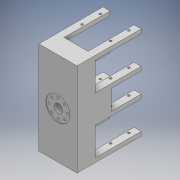
# Autodesk Inventor part: shoulder_5
Saved by Autodesk Inventor 2018 (Build 220112000, 112)
## iProperties
Created: 2020-10-13
Part Number: shoulder_5
Material: 일반
Document SubType Name: Sheet Metal
Designer: j3jjj
Density: 1 g/cm^3
Sheet Metal Rule: 기본값_mm
Appearance: 기본값
Author: j3jjj
Autodesk Inventor part; units mm, degrees
ref_plane "YZ Plane" through (0, 0, 0) normal (1, 0, 0) x (0, 1, 0)
ref_plane "XZ Plane" through (0, 0, 0) normal (0, 1, 0) x (-1, 0, 0)
ref_plane "XY Plane" through (0, 0, 0) normal (0, 0, 1) x (1, 0, 0)
sketch "스케치1" plane through (0, 0, 0) normal (0, 1, 0) x (-1, 0, 0)
  line L0 (23, -56) -> (-23, -56)
  line L1 (-23, -56) -> (-23, 56)
  line L2 (-23, 56) -> (23, 56)
  line L3 (23, 56) -> (23, -56)
  point P0 (0, 0)
  dimension "d0" = 112
  dimension "d1" = 56
  dimension "d2" = 46
  dimension "d3" = 23
  constraints: 8 end point, 2 parallel, 1 horizontal, 1 perpendicular
  measures "d0" distance between parallel lines of L0 L2
  measures "d1" distance from line of point (0, 0) L2
  measures "d2" distance between parallel lines of L1 L3
  measures "d3" distance from line of point (0, 0) L3
extrude "돌출1" add sketch "스케치1" along normal blind 16.1
sketch "스케치2" plane through (0, 0, 0) normal (0, -1, 0) x (1, 0, 0)
  circle A0 centre (0, 0) radius 14.52
  dimension "d6" = 29.04
  constraints: 1 centre point, 1 coincident
  measures "d6" diameter of A0
extrude "돌출2" cut sketch "스케치2" against normal blind 0.5
sketch "스케치3" plane through (0, 0.5, 0) normal (0, -1, 0) x (1, 0, 0)
  circle A0 centre (0, 0) radius 5.075
  circle A1 centre (0, 11) radius 1.25
  circle A2 centre (-7.7782, 7.7782) radius 1.25
  circle A3 centre (-11, 0) radius 1.25
  circle A4 centre (-7.7782, -7.7782) radius 1.25
  circle A5 centre (0, -11) radius 1.25
  circle A6 centre (7.7782, -7.7782) radius 1.25
  circle A7 centre (11, 0) radius 1.25
  circle A8 centre (7.7782, 7.7782) radius 1.25
  dimension "d9" = 10.15
  dimension "d10" = 2.5
  dimension "d11" = 11
  dimension "d14" = 360
  constraints: 9 centre point, 1 coincident, 17 other
  measures "d9" diameter of A0
  measures "d10" diameter of A1
  measures "d11" distance of point (0, 0) A1.centre
extrude "돌출3" cut sketch "스케치3" against normal blind 30
sketch "스케치4" plane through (0, 16.1, 0) normal (0, 1, 0) x (1, 0, 0)
  circle A0 centre (0, -11) radius 1.25 projected
  circle A1 centre (0, -11) radius 3
  circle A2 centre (7.7782, -7.7782) radius 3
  circle A3 centre (11, 0) radius 3
  circle A4 centre (7.7782, 7.7782) radius 3
  circle A5 centre (0, 11) radius 3
  circle A6 centre (-7.7782, 7.7782) radius 3
  circle A7 centre (-11, 0) radius 3
  circle A8 centre (-7.7782, -7.7782) radius 3
  point P0 (0, 0)
  dimension "d18" = 6
  dimension "d21" = 360
  constraints: 8 centre point, 1 coincident, 17 other
  measures "d18" diameter of A1
extrude "돌출4" cut sketch "스케치4" against normal blind 5 contours A0 | A1 | A2 | A3 | A4 | A5 | A6 | A7 | A8
sketch "스케치5" plane through (0, 16.1, 0) normal (0, 1, 0) x (1, 0, 0)
  line L0 (-23, -56) -> (23, -56)
  line L1 (23, -56) -> (23, -51)
  line L2 (23, -51) -> (-23, -51)
  line L3 (-23, -51) -> (-23, -56)
  line L4 (-23, -56) -> (23, -56) projected
  line L5 (-14.52, -51) -> (14.52, -51)
  line L6 (14.52, -51) -> (14.52, -56)
  line L7 (14.52, -56) -> (-14.52, -56)
  line L8 (-14.52, -56) -> (-14.52, -51)
  line L9 (0, 0) -> (-19.344, 0)
  line L10 (-23, 56) -> (23, 56)
  line L11 (23, 56) -> (23, 51)
  line L12 (23, 51) -> (-23, 51)
  line L13 (-23, 51) -> (-23, 56)
  line L14 (-23, 56) -> (23, 56)
  line L15 (-14.52, 51) -> (14.52, 51)
  line L16 (14.52, 51) -> (14.52, 56)
  line L17 (14.52, 56) -> (-14.52, 56)
  line L18 (-14.52, 56) -> (-14.52, 51)
  point P0 (-23, 56)
  dimension "d25" = 5
  dimension "d27" = 29.04
  dimension "d28" = 14.52
  constraints: 36 end point, 9 symmetric about line, 4 parallel, 4 point on line, 3 horizontal, 2 perpendicular
  measures "d25" distance between parallel lines of L2 L0
  measures "d27" distance between parallel lines of L6 L8
  measures "d28" distance from line of L9.start L8
extrude "돌출5" add sketch "스케치5" along normal blind 61.1 contours L3 L2 L8 L0 | L6 L2 L1 L0 | L10 L18 L12 L13 | L10 L11 L12 L16
sketch "스케치6" plane through (0, 16.1, 0) normal (0, 1, 0) x (1, 0, 0)
  line L0 (-23, -56) -> (-23, 56) projected
  line L1 (-23, -16.98) -> (-14.52, -16.98)
  line L2 (-14.52, 16.98) -> (-23, 16.98)
  line L3 (-14.52, -51) -> (-23, -51) projected
  line L4 (-23, 51) -> (-14.52, 51) projected
  line L5 (-23, -16.98) -> (-14.52, -16.98)
  line L6 (-14.52, -16.98) -> (-14.52, -11.98)
  line L7 (-14.52, -11.98) -> (-23, -11.98)
  line L8 (-23, -11.98) -> (-23, -16.98)
  line L9 (-23, 16.98) -> (-14.52, 16.98)
  line L10 (-14.52, 16.98) -> (-14.52, 11.98)
  line L11 (-14.52, 11.98) -> (-23, 11.98)
  line L12 (-23, 11.98) -> (-23, 16.98)
  circle A0 centre (0, 0) radius 14.52 projected
  line L13 (0, 0) -> (0, -35.0493)
  line L14 (23, -16.98) -> (14.52, -16.98)
  line L15 (14.52, 16.98) -> (23, 16.98)
  line L16 (23, -16.98) -> (14.52, -16.98)
  line L17 (14.52, -16.98) -> (14.52, -11.98)
  line L18 (14.52, -11.98) -> (23, -11.98)
  line L19 (23, -11.98) -> (23, -16.98)
  line L20 (23, 16.98) -> (14.52, 16.98)
  line L21 (14.52, 16.98) -> (14.52, 11.98)
  line L22 (14.52, 11.98) -> (23, 11.98)
  line L23 (23, 11.98) -> (23, 16.98)
  dimension "d31" = 34.02
  dimension "d32" = 34.02
  dimension "d34" = 5
  dimension "d35" = 5
  dimension "d36" = 8.48
  dimension "d37" = 8.48
  constraints: 42 end point, 10 symmetric about line, 5 parallel, 3 horizontal, 2 perpendicular, 1 point on line, 1 vertical
  measures "d31" distance between parallel lines of L1 L3
  measures "d32" distance between parallel lines of L4 L2
  measures "d34" distance of L6.end L5.end
  measures "d35" distance of L9.end L10.end
  measures "d36" distance between parallel lines of L6 L0
  measures "d37" distance between parallel lines of L10 L0
extrude "돌출6" add sketch "스케치6" along normal blind 61.1 contours L0 L2 L10 L11 | L0 L7 L6 L1 | L14 L17 L18 L19 | L15 L23 L22 L21
sketch "스케치7" plane through (0, 16.1, 0) normal (0, 1, 0) x (1, 0, 0)
  line L0 (-14.52, -51) -> (-14.52, -56) projected
  line L1 (14.52, -51) -> (23, -51) projected
  line L2 (-14.52, -56) -> (14.52, -56)
  line L3 (14.52, -56) -> (14.52, -51)
  line L4 (14.52, -51) -> (-14.52, -51)
  line L5 (-14.52, -51) -> (-14.52, -56)
  line L6 (-14.52, 51) -> (-23, 51) projected
  line L7 (14.52, 51) -> (14.52, 56) projected
  line L8 (-14.52, 51) -> (14.52, 51)
  line L9 (14.52, 51) -> (14.52, 56)
  line L10 (14.52, 56) -> (-14.52, 56)
  line L11 (-14.52, 56) -> (-14.52, 51)
  line L12 (-23, -16.98) -> (-23, -51) projected
  line L13 (-23, -16.98) -> (-14.52, -16.98) projected
  line L14 (-23, -51) -> (-20, -51)
  line L15 (-20, -51) -> (-20, -16.98)
  line L16 (-20, -16.98) -> (-23, -16.98)
  line L17 (-23, -16.98) -> (-23, -51)
  line L18 (-23, 16.98) -> (-14.52, 16.98) projected
  line L19 (-23, 16.98) -> (-20, 16.98)
  line L20 (-20, 16.98) -> (-20, 51)
  line L21 (-20, 51) -> (-23, 51)
  line L22 (-23, 51) -> (-23, 16.98)
  line L23 (23, 56) -> (23, -56) projected
  line L24 (23, 51) -> (20, 51)
  line L25 (20, 51) -> (20, 16.98)
  line L26 (20, 16.98) -> (23, 16.98)
  line L27 (23, 16.98) -> (23, 51)
  line L28 (23, -51) -> (23, -16.98) projected
  line L29 (23, -16.98) -> (20, -16.98)
  line L30 (20, -16.98) -> (20, -51)
  line L31 (20, -51) -> (23, -51)
  line L32 (23, -51) -> (23, -16.98)
  point P0 (0, 0)
  dimension "d40" = 3
  dimension "d41" = 3
  dimension "d42" = 3
  dimension "d43" = 3
  constraints: 48 end point, 12 parallel, 6 horizontal, 6 perpendicular, 6 point on line
  measures "d40" distance of L16.end L15.end
  measures "d41" distance of L21.end L20.end
  measures "d42" distance of L26.end L25.end
  measures "d43" distance of L31.end L30.end
extrude "돌출7" add sketch "스케치7" along normal blind 5.6
sketch "스케치8" plane through (0, 16.1, 0) normal (0, 1, 0) x (1, 0, 0)
  line L0 (23, 11.98) -> (14.52, 11.98) projected
  line L1 (23, -11.98) -> (14.52, -11.98)
  line L2 (14.52, -11.98) -> (14.52, 11.98)
  line L3 (14.52, 11.98) -> (23, 11.98)
  line L4 (23, 11.98) -> (23, -11.98)
  line L5 (-23, 11.98) -> (-23, -11.98) projected
  line L6 (-14.52, -11.98) -> (-14.52, -16.98) projected
  line L7 (-23, 11.98) -> (-14.52, 11.98)
  line L8 (-14.52, 11.98) -> (-14.52, -11.98)
  line L9 (-14.52, -11.98) -> (-23, -11.98)
  line L10 (-23, -11.98) -> (-23, 11.98)
  point P0 (0, 0)
  constraints: 16 end point, 4 parallel, 2 horizontal, 2 perpendicular
extrude "돌출8" add sketch "스케치8" along normal blind 25
sketch "스케치9" plane through (-23, 0, 56) normal (0, 0, 1) x (1, 0, 0)
  circle A0 centre (5.8, 68.2) radius 1.35
  line L0 (0, 77.2) -> (8.48, 77.2) projected
  line L1 (0, 0) -> (0, 77.2) projected
  circle A1 centre (5.8, 46.2) radius 1.35
  line L2 (23, 0) -> (23, 16.9494)
  circle A2 centre (40.2, 68.2) radius 1.35
  circle A3 centre (40.2, 46.2) radius 1.35
  dimension "d48" = 9
  dimension "d49" = 5.8
  dimension "d50" = 22
  dimension "d51" = 2.7
  dimension "d52" = 2.7
  dimension "d53" = 5.8
  constraints: 4 centre point, 2 end point, 2 symmetric about line, 1 vertical, 2 other
  measures "d48" distance from line of A0.centre L0
  measures "d49" distance from line of A0.centre L1
  measures "d50" distance of A0.centre A1.centre
  measures "d51" diameter of A1
  measures "d52" diameter of A0
  measures "d53" distance from line of A1.centre L1
extrude "돌출9" cut sketch "스케치9" against normal blind 300
equation "\"TransitionRadius\" = BendRadius"
equation "\"BendRadius\" = 0.5"
